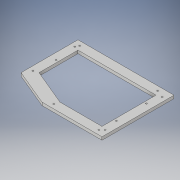
# Autodesk Inventor part: Panel
Saved by Autodesk Inventor 2018 (Build 220112000, 112)
## iProperties
Created: 2018-10-20
Part Number: Panel
Material: Generic
Document SubType Name: Modeling
Designer: jpark
Density: 1 g/cm^3
Appearance: Default
Author: jpark
Autodesk Inventor part; units mm, degrees
ref_plane "YZ Plane" through (0, 0, 0) normal (1, 0, 0) x (0, 1, 0)
ref_plane "XZ Plane" through (0, 0, 0) normal (0, 1, 0) x (-1, 0, 0)
ref_plane "XY Plane" through (0, 0, 0) normal (0, 0, 1) x (1, 0, 0)
sketch "Sketch1" plane through (0, 0, 0) normal (0, 1, 0) x (-1, 0, 0)
  line L0 (0, 0) -> (0, -152.4)
  line L1 (0, -152.4) -> (203.2, -152.4)
  line L2 (203.2, -152.4) -> (203.2, -31.75)
  line L3 (203.2, -31.75) -> (127, 0)
  line L4 (127, 0) -> (0, 0)
  dimension "d0" = 120.65
  dimension "d1" = 203.2
  dimension "d2" = 127
  dimension "d3" = 152.4
  constraints: 10 end point, 3 perpendicular, 1 vertical
  measures "d0" distance of L1.end L2.end
  measures "d1" distance of L0.end L1.end
  measures "d2" distance of L3.end L0.start
  measures "d3" distance of L0.start L0.end
extrude "Extrusion1" add sketch "Sketch1" along normal blind 6.35
sketch "Sketch3" plane through (0, 6.35, 0) normal (0, 1, 0) x (1, 0, 0)
  line L0 (0, 0) -> (0, 152.4) projected
  line L1 (0, 152.4) -> (-203.2, 152.4) projected
  line L2 (-203.2, 152.4) -> (-203.2, 31.75) projected
  line L3 (-203.2, 31.75) -> (-127, 0) projected
  line L4 (-127, 0) -> (0, 0) projected
  line L5 (-19.05, 19.05) -> (-19.05, 133.35)
  line L6 (-19.05, 133.35) -> (-184.15, 133.35)
  line L7 (-184.15, 133.35) -> (-184.15, 50.8)
  line L8 (-19.05, 19.05) -> (-107.95, 19.05)
  line L9 (-107.95, 19.05) -> (-184.15, 50.8)
  circle A0 centre (-9.271, 15.875) radius 1.524
  circle A1 centre (-9.271, 136.525) radius 1.524
  circle A2 centre (-25.4, 143.129) radius 1.524
  circle A3 centre (-190.5, 143.129) radius 1.524
  circle A4 centre (-193.929, 47.625) radius 1.524
  circle A5 centre (-193.929, 136.525) radius 1.524
  circle A6 centre (-15.875, 9.271) radius 1.524
  circle A7 centre (-111.125, 9.271) radius 1.524
  dimension "d10" = 120.65
  dimension "d11" = 82.55
  dimension "d12" = 203.2
  dimension "d13" = 165.1
  dimension "d14" = 114.3
  dimension "d15" = 88.9
  dimension "d16" = 19.05
  dimension "d17" = 19.05
  dimension "d18" = 3.048
  dimension "d19" = 3.048
  dimension "d20" = 120.65
  dimension "d21" = 3.048
  dimension "d22" = 3.048
  dimension "d23" = 15.875
  dimension "d24" = 9.271
  dimension "d25" = 9.271
  dimension "d26" = 9.271
  dimension "d27" = 25.4
  dimension "d28" = 12.7
  dimension "d29" = 9.271
  dimension "d30" = 3.048
  dimension "d31" = 3.048
  dimension "d32" = 88.9
  dimension "d33" = 15.875
  dimension "d34" = 9.271
  dimension "d35" = 9.271
  dimension "d36" = 3.048
  dimension "d37" = 9.271
  dimension "d38" = 15.875
  dimension "d39" = 3.048
  dimension "d40" = 15.875
  dimension "d41" = 9.271
  constraints: 10 end point, 8 centre point, 2 perpendicular, 1 horizontal, 1 vertical
  measures "d10" distance of L1.end L2.end
  measures "d11" distance of L6.end L7.end
  measures "d12" distance of L0.end L1.end
  measures "d13" distance of L5.end L6.end
  measures "d14" distance of L5.start L5.end
  measures "d15" distance of L5.start L8.end
  measures "d16" distance between parallel lines of L1 L6
  measures "d17" distance between parallel lines of L2 L7
  measures "d18" diameter of A0
  measures "d19" diameter of A1
  measures "d20" distance of A1.centre A0.centre
  measures "d21" diameter of A2
  measures "d22" diameter of A3
  measures "d23" vertical distance of L0.end A1.centre
  measures "d24" distance from line of L0 A1.centre
  measures "d25" distance from line of L0 A0.centre
  measures "d26" distance from line of L1 A2.centre
  measures "d27" distance from line of L0 A2.centre
  measures "d28" distance from line of L2 A3.centre
  measures "d29" distance from line of L1 A3.centre
  measures "d30" diameter of A4
  measures "d31" diameter of A5
  measures "d32" distance of A5.centre A4.centre
  measures "d33" vertical distance of L2.end A4.centre
  measures "d34" distance from line of L2 A4.centre
  measures "d35" distance from line of L2 A5.centre
  measures "d36" diameter of A6
  measures "d37" vertical distance of point (0, 0) A6.centre
  measures "d38" horizontal distance of point (0, 0) A6.centre
  measures "d39" diameter of A7
  measures "d40" horizontal distance of L3.end A7.centre
  measures "d41" vertical distance of L3.end A7.centre
extrude "Extrusion2" cut sketch "Sketch3" against normal blind 6.35 contours L8 L9 L7 L6 L5 | A0 | A1 | A2 | A3 | A4 | A5 | A6 | A7
sketch "Sketch4" plane through (0, 6.35, 0) normal (0, 1, 0) x (1, 0, 0)
  circle A0 centre (-13.97, 44.45) radius 1.524
  circle A1 centre (-13.97, 107.95) radius 1.524
  circle A2 centre (-189.23, 92.075) radius 1.524
  line L0 (-107.95, 19.05) -> (-184.15, 50.8) projected
  line L1 (-184.15, 50.8) -> (-184.15, 133.35) projected
  line L2 (-19.05, 133.35) -> (-19.05, 19.05) projected
  point P0 (0, 0)
  dimension "d44" = 3.048
  dimension "d45" = 3.048
  dimension "d46" = 3.048
  dimension "d47" = 82.55
  dimension "d48" = 41.275
  dimension "d49" = 5.08
  dimension "d50" = 25.4
  dimension "d51" = 25.4
  dimension "d52" = 5.08
  dimension "d53" = 5.08
  constraints: 3 centre point
  measures "d44" diameter of A0
  measures "d45" diameter of A1
  measures "d46" diameter of A2
  measures "d47" distance of L0.end L1.end
  measures "d48" vertical distance of L0.end A2.centre
  measures "d49" distance from line of L1 A2.centre
  measures "d50" vertical distance of L2.start A1.centre
  measures "d51" vertical distance of L2.end A0.centre
  measures "d52" distance from line of L2 A0.centre
  measures "d53" distance from line of L2 A1.centre
extrude "Extrusion3" cut sketch "Sketch4" against normal blind 6.35
body "Solid1"
